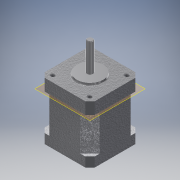
# Autodesk Inventor part: nema 17 stepper motor (triple stack)
Saved by Autodesk Inventor 2017 (Build 210142000, 142)
## iProperties
Created: 2013-12-03
Part Number: nema 17 stepper motor (triple stack)
Material: Generic
Document SubType Name: Modeling
Designer: Samoray
Density: 1 g/cm^3
Appearance: Default
Author: Samoray
Autodesk Inventor part; units mm, degrees
ref_plane "YZ Plane" through (0, 0, 0) normal (1, 0, 0) x (0, 1, 0)
ref_plane "XZ Plane" through (0, 0, 0) normal (0, 1, 0) x (-1, 0, 0)
ref_plane "XY Plane" through (0, 0, 0) normal (0, 0, 1) x (1, 0, 0)
sketch "Sketch1" plane through (0, 0, 0) normal (0, 0, 1) x (1, 0, 0)
  line L0 (21, 42) -> (-21, 42)
  line L1 (-21, 42) -> (-21, 0)
  line L2 (-21, 0) -> (21, 0)
  line L3 (21, 0) -> (21, 42)
  point P0 (0, 0)
  point P1 (0, 0)
  dimension "d0" = 42
  dimension "d1" = 42
  constraints: 8 end point, 2 parallel, 1 coincident, 1 horizontal, 1 midpoint, 1 perpendicular
  measures "d0" distance of L0.end L1.end
  measures "d1" distance of L0.start L0.end
extrude "Extrusion1" add sketch "Sketch1" along normal blind 48
ref_plane "Work Plane1" through (0, 0, 38) normal (0, 0, 1) x (1, 0, 0)
sketch "Sketch2" plane through (0, 0, 38) normal (0, 0, 1) x (1, 0, 0)
  line L0 (21, 42) -> (-21, 42)
  line L1 (-21, 42) -> (-21, 0)
  line L2 (-21, 0) -> (21, 0)
  line L3 (21, 0) -> (21, 42)
  line L4 (-21, 42) -> (-21, 0) projected
  line L5 (-21, 34) -> (-13, 42)
  line L6 (21, 42) -> (-21, 42) projected
  line L7 (0, 50.0167) -> (0, -8.0167)
  line L8 (-21, 21) -> (21, 21)
  line L9 (21, 34) -> (13, 42)
  line L10 (-21, 8) -> (-13, 0)
  line L11 (21, 8) -> (13, 0)
  line L12 (-21, 34) -> (-21, 42)
  line L13 (-13, 42) -> (-21, 42)
  line L14 (13, 42) -> (21, 42)
  line L15 (21, 42) -> (21, 34)
  line L16 (21, 8) -> (21, 0)
  line L17 (21, 0) -> (21, 42) projected
  line L18 (-21, 0) -> (21, 0) projected
  line L19 (21, 0) -> (13, 0)
  line L20 (-13, 0) -> (-21, 0)
  line L21 (-21, 0) -> (-21, 8)
  point P0 (0, 0)
  point P1 (0, 21)
  dimension "d5" = 8
  dimension "d6" = 8
  dimension "d7" = 42
  constraints: 36 end point, 6 symmetric about line, 4 collinear, 4 midpoint, 4 perpendicular, 4 point on line, 2 parallel, 1 horizontal
  measures "d5" distance of L0.end L5.start
  measures "d6" distance of L0.end L5.end
  measures "d7" diameter of L0 L8
extrude "Extrusion2" cut sketch "Sketch2" against normal blind 30 contours L3 L9 L0 | L5 L1 L0 | L3 L2 L11 | L2 L1 L10
chamfer "Chamfer1" distance 4 angle 45 8 edges at (-21, 42, 43) (21, 42, 43) (21, 0, 43) (-21, 0, 43) (-21, 42, 4) (21, 42, 4) (-21, 0, 4) (21, 0, 4)
sketch "Sketch3" plane through (0, 0, 48) normal (0, 0, 1) x (1, 0, 0)
  line L0 (21, 38) -> (21, 4) projected
  line L1 (-17, 42) -> (17, 42) projected
  line L2 (-21, 4) -> (-21, 38) projected
  line L3 (0, 42) -> (0, 0)
  line L4 (-21, 21) -> (21, 21)
  point P0 (-15.5, 5.5)
  point P1 (15.5, 5.5)
  point P2 (-15.5, 36.5)
  point P3 (15.5, 36.5)
  dimension "d13" = 31
  dimension "d14" = 31
  constraints: 4 end point, 3 midpoint, 3 symmetric about line, 1 parallel
  measures "d13" diameter of point (-15.5, 5.5) L3
  measures "d14" diameter of point (-15.5, 5.5) L4
hole "Hole1" at (-15.5, 5.5, 48) at (15.5, 5.5, 48) at (-15.5, 36.5, 48) at (15.5, 36.5, 48) direction (0, 0, -1) diameter 3 depth 4.5 tip angle 118 countersink diameter 4 countersink angle 90
sketch "Sketch5" plane through (0, 0, 0) normal (0, 0, -1) x (-1, 0, 0)
  line L0 (17, 0) -> (-17, 0) projected
  line L1 (17, 42) -> (-17, 42) projected
  line L2 (0, 42) -> (0, 0)
  point P0 (-9.5, 21)
  point P1 (9.5, 21)
  dimension "d28" = 19
  constraints: 2 end point, 1 midpoint, 1 perpendicular, 1 symmetric about line
  measures "d28" diameter of point (-9.5, 21) L2
hole "Hole2" at (9.5, 21, 0) at (-9.5, 21, 0) direction (0, 0, 1) diameter 2 depth 5.1 tip angle 118
sketch "Sketch6" plane through (0, 0, 48) normal (0, 0, 1) x (1, 0, 0)
  line L0 (-17, 42) -> (17, 42) projected
  line L1 (-21, 4) -> (-21, 38) projected
  line L2 (0, 42) -> (0, 0)
  circle A0 centre (0, 21) radius 11
  dimension "d36" = 22
  constraints: 2 end point, 2 midpoint, 1 centre point, 1 parallel
  measures "d36" diameter of A0
extrude "Extrusion4" add sketch "Sketch6" along normal blind 2.03
fillet "Fillet1" radius 0.7 1 edges at (-11, 21, 48)
sketch "Sketch7" plane through (0, 21, 50.03) normal (0, 0, 1) x (1, 0, 0)
  circle A0 centre (0, 0) radius 11 projected
  circle A1 centre (0, 0) radius 2.5
  point P0 (0, -21)
  dimension "d40" = 5
  constraints: 1 centre point, 1 coincident
  measures "d40" diameter of A1
extrude "Extrusion5" add sketch "Sketch7" along normal blind 23.88 contours A1
sketch "Sketch8" plane through (0, 21, 73.91) normal (0, 0, 1) x (1, 0, 0)
  line L0 (-1.473, 2.02) -> (1.473, 2.02)
  circle A0 centre (0, 0) radius 2.5 projected
  circle A1 centre (0, 0) radius 2.5 projected
  circle A2 centre (0, 0) radius 2.5 projected
  arc A3 (1.473, 2.02) -> (-1.473, 2.02) centre (0, 0) ccw
  point P0 (0, -21)
  constraints: 2 end point, 2 point on circle, 1 centre point, 1 coincident, 1 horizontal
extrude "Extrusion6" cut sketch "Sketch8" against normal blind 14.86 contours A0 L0 picked at (0.3249, 2.2492)
chamfer "Chamfer2" distance 0.5 angle 45 2 edges at (-1.1331, 18.7715, 73.91) (2.2285, 22.1331, 73.91)
body "Solid1"
